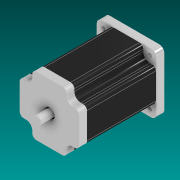
# Autodesk Inventor part: Nema 23 High toque
Saved by Autodesk Inventor 2020.3 (Build 243373000, 373)
## iProperties
Created: 2020-05-18
Part Number: Nema 23 High toque
Material: Aluminum 6061
Document SubType Name: Modeling
Designer: Svend
Density: 2.7 g/cm^3
Appearance: Aluminum - Polished
Author: Svend
Autodesk Inventor part; units mm, degrees
ref_plane "YZ Plane" through (0, 0, 0) normal (1, 0, 0) x (0, 1, 0)
ref_plane "XZ Plane" through (0, 0, 0) normal (0, 1, 0) x (-1, 0, 0)
ref_plane "XY Plane" through (0, 0, 0) normal (0, 0, 1) x (1, 0, 0)
sketch "Sketch1" plane through (0, 0, 0) normal (0, 0, 1) x (1, 0, 0)
  line L0 (24.95, 29.95) -> (-24.95, 29.95)
  line L1 (-29.95, 24.95) -> (-29.95, -24.95)
  line L2 (-24.95, -29.95) -> (24.95, -29.95)
  line L3 (29.95, -24.95) -> (29.95, 24.95)
  line L4 (29.95, 29.95) -> (-29.95, -29.95) construction
  line L5 (-29.95, 29.95) -> (29.95, -29.95) construction
  circle A0 centre (-23.57, 23.57) radius 2
  circle A1 centre (23.57, 23.57) radius 2
  circle A2 centre (23.57, -23.57) radius 2
  circle A3 centre (-23.57, -23.57) radius 2
  circle A4 centre (0, 0) radius 4.5
  arc A5 (-24.95, 29.95) -> (-29.95, 24.95) centre (-24.95, 24.95) ccw
  arc A6 (29.95, 24.95) -> (24.95, 29.95) centre (24.95, 24.95) ccw
  arc A7 (24.95, -29.95) -> (29.95, -24.95) centre (24.95, -24.95) ccw
  arc A8 (-29.95, -24.95) -> (-24.95, -29.95) centre (-24.95, -24.95) ccw
  dimension "d0" = 59.9
  dimension "d2" = 47.14
  dimension "d3" = 47.14
  dimension "d4" = 4
  dimension "d5" = 9
  dimension "d6" = 5
  dimension "d7" = 59.9
  dimension "d8" = 5
  dimension "d9" = 5
  constraints: 12 end point, 12 point on line, 9 centre point, 8 point on circle, 8 tangent, 4 equal radius, 2 horizontal alignment, 2 midpoint, 2 parallel, 1 coincident, 1 horizontal, 1 perpendicular
  measures "d0" distance of L5.end L4.end
  measures "d2" distance of A0.centre A1.centre
  measures "d3" distance of A2.centre A1.centre
  measures "d4" diameter of A0
  measures "d5" diameter of A4
  measures "d6" radius of A5
  measures "d7" distance between parallel lines of L2 L0
  measures "d8" radius of A6
  measures "d9" radius of A7
extrude "Extrusion1" add sketch "Sketch1" along normal blind 8
chamfer "Chamfer1" distance 0.5 angle 45 4 edges at (21.57, -23.57, 0) (-25.57, -23.57, 0) (21.57, 23.57, 0) (-25.57, 23.57, 0)
sketch "Sketch2" plane through (0, 0, 0) normal (0, 0, -1) x (-1, 0, 0)
  circle A0 centre (0, 0) radius 5 projected
  circle A1 centre (0, 0) radius 19
  circle A2 centre (0, 0) radius 4.5 projected
  dimension "d23" = 38
  constraints: 1 centre point, 1 coincident
  measures "d23" diameter of A1
extrude "Extrusion2" add sketch "Sketch2" along normal blind 2 contours A0 | A1
chamfer "Chamfer2" distance 0.5 angle 45 2 edges at (4.5, 0, -2) (19, 0, -2)
sketch "Sketch3" plane through (0, 0, 8) normal (0, 0, 1) x (1, 0, 0)
  arc A0 (24.95, -29.95) -> (29.95, -24.95) centre (24.95, -24.95) ccw projected
  line L0 (29.95, -24.95) -> (29.95, 24.95) projected
  arc A1 (29.95, 24.95) -> (24.95, 29.95) centre (24.95, 24.95) ccw projected
  line L1 (24.95, 29.95) -> (-24.95, 29.95) projected
  arc A2 (-24.95, 29.95) -> (-29.95, 24.95) centre (-24.95, 24.95) ccw projected
  line L2 (-29.95, 24.95) -> (-29.95, -24.95) projected
  arc A3 (-29.95, -24.95) -> (-24.95, -29.95) centre (-24.95, -24.95) ccw projected
  line L3 (-24.95, -29.95) -> (24.95, -29.95) projected
  circle A4 centre (0, 0) radius 4.5 projected
  circle A5 centre (-23.57, 23.57) radius 2 projected
  circle A6 centre (23.57, -23.57) radius 2 projected
  circle A7 centre (-23.57, -23.57) radius 2 projected
  circle A8 centre (23.57, 23.57) radius 2 projected
  circle A9 centre (-23.57, -23.57) radius 2 projected
  circle A10 centre (-23.57, -23.57) radius 6.38
  line L4 (-29.95, 24.95) -> (-29.95, -24.95) projected
  circle A11 centre (-23.57, 23.57) radius 2 projected
  circle A12 centre (-23.57, 23.57) radius 6.38
  line L5 (24.95, 29.95) -> (-24.95, 29.95) projected
  circle A13 centre (23.57, 23.57) radius 2 projected
  circle A14 centre (23.57, 23.57) radius 6.38
  circle A15 centre (23.57, -23.57) radius 6.38
  line L6 (-24.95, -29.95) -> (24.95, -29.95) projected
  line L7 (23.57, -17.19) -> (25.95, -17.19)
  line L8 (29.95, -24.95) -> (29.95, 24.95) projected
  line L9 (17.19, -23.57) -> (17.19, -25.95)
  line L10 (-17.19, -23.57) -> (-17.19, -25.95)
  line L11 (-23.57, -17.19) -> (-25.95, -17.19)
  line L12 (-23.57, 17.19) -> (-25.95, 17.19)
  line L13 (-17.19, 23.57) -> (-17.19, 25.95)
  line L14 (17.19, 23.57) -> (17.19, 25.95)
  line L15 (23.57, 17.19) -> (25.95, 17.19)
  line L16 (24.95, 29.95) -> (-24.95, 29.95) projected
  line L17 (29.95, -24.95) -> (29.95, 24.95) projected
  line L18 (-13.19, -29.95) -> (13.19, -29.95)
  line L19 (29.95, -13.19) -> (29.95, 13.19)
  line L20 (13.19, 29.95) -> (-13.19, 29.95)
  line L21 (-29.95, 13.19) -> (-29.95, -13.19)
  arc A16 (-29.95, -13.19) -> (-25.95, -17.19) centre (-25.95, -13.19) ccw
  arc A17 (-25.95, 17.19) -> (-29.95, 13.19) centre (-25.95, 13.19) ccw
  arc A18 (-13.19, 29.95) -> (-17.19, 25.95) centre (-13.19, 25.95) ccw
  arc A19 (17.19, 25.95) -> (13.19, 29.95) centre (13.19, 25.95) ccw
  arc A20 (29.95, 13.19) -> (25.95, 17.19) centre (25.95, 13.19) ccw
  arc A21 (25.95, -17.19) -> (29.95, -13.19) centre (25.95, -13.19) ccw
  arc A22 (13.19, -29.95) -> (17.19, -25.95) centre (13.19, -25.95) ccw
  arc A23 (-17.19, -25.95) -> (-13.19, -29.95) centre (-13.19, -25.95) ccw
  point P0 (29.95, -17.19)
  point P1 (17.19, -29.95)
  point P2 (-17.19, -29.95)
  point P3 (-29.95, -17.19)
  point P4 (-29.95, 17.19)
  point P5 (-17.19, 29.95)
  point P6 (17.19, 29.95)
  point P7 (29.95, 17.19)
  point P8 (29.95, 13.19)
  dimension "d29" = 4
  dimension "d30" = 4
  constraints: 28 tangent, 24 end point, 24 point on circle, 24 point on line, 12 centre point, 7 parallel, 6 equal radius, 6 perpendicular, 4 coincident, 3 collinear, 2 horizontal, 1 vertical
  measures "d29" radius of A16
  measures "d30" radius of A23
extrude "Extrusion3" add sketch "Sketch3" along normal blind 70 contours L3 A23 L10 A10 L11 A16 L2 A17 L12 A12 L13 A18 L1 A19 L14 A14 L15 A20 L0 A21 L7 A15 L9 A22
sketch "Sketch5" plane through (0, 0, 78) normal (0, 0, 1) x (1, 0, 0)
  arc A0 (17.19, 23.57) -> (23.57, 17.19) centre (23.57, 23.57) ccw projected
  line L0 (17.19, 23.57) -> (17.19, 25.95) projected
  arc A1 (17.19, 25.95) -> (13.19, 29.95) centre (13.19, 25.95) ccw projected
  line L1 (13.19, 29.95) -> (-13.19, 29.95) projected
  arc A2 (-13.19, 29.95) -> (-17.19, 25.95) centre (-13.19, 25.95) ccw projected
  line L2 (-17.19, 25.95) -> (-17.19, 23.57) projected
  arc A3 (-23.57, 17.19) -> (-17.19, 23.57) centre (-23.57, 23.57) ccw projected
  line L3 (-23.57, 17.19) -> (-25.95, 17.19) projected
  arc A4 (-25.95, 17.19) -> (-29.95, 13.19) centre (-25.95, 13.19) ccw projected
  line L4 (-29.95, 13.19) -> (-29.95, -13.19) projected
  arc A5 (-29.95, -13.19) -> (-25.95, -17.19) centre (-25.95, -13.19) ccw projected
  line L5 (-25.95, -17.19) -> (-23.57, -17.19) projected
  arc A6 (-17.19, -23.57) -> (-23.57, -17.19) centre (-23.57, -23.57) ccw projected
  line L6 (-17.19, -23.57) -> (-17.19, -25.95) projected
  arc A7 (-17.19, -25.95) -> (-13.19, -29.95) centre (-13.19, -25.95) ccw projected
  line L7 (-13.19, -29.95) -> (13.19, -29.95) projected
  arc A8 (13.19, -29.95) -> (17.19, -25.95) centre (13.19, -25.95) ccw projected
  line L8 (17.19, -25.95) -> (17.19, -23.57) projected
  arc A9 (23.57, -17.19) -> (17.19, -23.57) centre (23.57, -23.57) ccw projected
  line L9 (23.57, -17.19) -> (25.95, -17.19) projected
  arc A10 (25.95, -17.19) -> (29.95, -13.19) centre (25.95, -13.19) ccw projected
  line L10 (29.95, -13.19) -> (29.95, 13.19) projected
  arc A11 (29.95, 13.19) -> (25.95, 17.19) centre (25.95, 13.19) ccw projected
  line L11 (25.95, 17.19) -> (23.57, 17.19) projected
  circle A12 centre (0, 0) radius 4.5 projected
  line L12 (-23.57, -17) -> (-25.95, -17)
  arc A13 (-29.76, -13.19) -> (-25.95, -17) centre (-25.95, -13.19) ccw
  line L13 (-29.76, -13.19) -> (-29.76, 13.19)
  arc A14 (-25.95, 17) -> (-29.76, 13.19) centre (-25.95, 13.19) ccw
  line L14 (-25.95, 17) -> (-23.57, 17)
  arc A15 (-23.57, 17) -> (-17, 23.57) centre (-23.57, 23.57) ccw
  line L15 (-17, 23.57) -> (-17, 25.95)
  arc A16 (-13.19, 29.76) -> (-17, 25.95) centre (-13.19, 25.95) ccw
  line L16 (-13.19, 29.76) -> (13.19, 29.76)
  arc A17 (17, 25.95) -> (13.19, 29.76) centre (13.19, 25.95) ccw
  line L17 (17, 25.95) -> (17, 23.57)
  arc A18 (17, 23.57) -> (23.57, 17) centre (23.57, 23.57) ccw
  line L18 (23.57, 17) -> (25.95, 17)
  arc A19 (29.76, 13.19) -> (25.95, 17) centre (25.95, 13.19) ccw
  line L19 (29.76, 13.19) -> (29.76, -13.19)
  arc A20 (25.95, -17) -> (29.76, -13.19) centre (25.95, -13.19) ccw
  line L20 (25.95, -17) -> (23.57, -17)
  arc A21 (23.57, -17) -> (17, -23.57) centre (23.57, -23.57) ccw
  line L21 (17, -23.57) -> (17, -25.95)
  arc A22 (13.19, -29.76) -> (17, -25.95) centre (13.19, -25.95) ccw
  line L22 (13.19, -29.76) -> (-13.19, -29.76)
  arc A23 (-17, -25.95) -> (-13.19, -29.76) centre (-13.19, -25.95) ccw
  line L23 (-17, -25.95) -> (-17, -23.57)
  arc A24 (-17, -23.57) -> (-23.57, -17) centre (-23.57, -23.57) ccw
  dimension "d38" = 0.19
  constraints: 24 end point, 24 point on circle, 12 centre point, 23 other
  measures "d38" distance between parallel lines of L5 L12
extrude "Extrusion6" cut sketch "Sketch5" against normal up to surface (70 mm away) contours A0 L11 A11 L10 A10 L9 A9 L8 A8 L7 A7 L6 A6 L5 A5 L4 A4 L3 A3 L2 A2 L1 A1 L0
sketch "Sketch6" plane through (0, 0, 78) normal (0, 0, 1) x (1, 0, 0)
  line L0 (25.95, 17) -> (23.57, 17) projected
  arc A0 (17, 23.57) -> (23.57, 17) centre (23.57, 23.57) ccw projected
  line L1 (17, 23.57) -> (17, 25.95) projected
  arc A1 (17, 25.95) -> (13.19, 29.76) centre (13.19, 25.95) ccw projected
  line L2 (13.19, 29.76) -> (-13.19, 29.76) projected
  arc A2 (-13.19, 29.76) -> (-17, 25.95) centre (-13.19, 25.95) ccw projected
  line L3 (-17, 25.95) -> (-17, 23.57) projected
  arc A3 (-23.57, 17) -> (-17, 23.57) centre (-23.57, 23.57) ccw projected
  line L4 (-23.57, 17) -> (-25.95, 17) projected
  arc A4 (-25.95, 17) -> (-29.76, 13.19) centre (-25.95, 13.19) ccw projected
  line L5 (-29.76, 13.19) -> (-29.76, -13.19) projected
  arc A5 (-29.76, -13.19) -> (-25.95, -17) centre (-25.95, -13.19) ccw projected
  line L6 (-25.95, -17) -> (-23.57, -17) projected
  arc A6 (-17, -23.57) -> (-23.57, -17) centre (-23.57, -23.57) ccw projected
  line L7 (-17, -23.57) -> (-17, -25.95) projected
  arc A7 (-17, -25.95) -> (-13.19, -29.76) centre (-13.19, -25.95) ccw projected
  line L8 (-13.19, -29.76) -> (13.19, -29.76) projected
  arc A8 (13.19, -29.76) -> (17, -25.95) centre (13.19, -25.95) ccw projected
  line L9 (17, -25.95) -> (17, -23.57) projected
  arc A9 (23.57, -17) -> (17, -23.57) centre (23.57, -23.57) ccw projected
  line L10 (23.57, -17) -> (25.95, -17) projected
  arc A10 (25.95, -17) -> (29.76, -13.19) centre (25.95, -13.19) ccw projected
  line L11 (29.76, -13.19) -> (29.76, 13.19) projected
  arc A11 (29.76, 13.19) -> (25.95, 17) centre (25.95, 13.19) ccw projected
  circle A12 centre (0, 0) radius 4.5 projected
  arc A13 (-29.902, -13.19) -> (-25.95, -17.142) centre (-25.95, -13.19) ccw
  line L12 (-29.902, -13.19) -> (-29.902, 13.19)
  arc A14 (-25.95, 17.142) -> (-29.902, 13.19) centre (-25.95, 13.19) ccw
  line L13 (-25.95, 17.142) -> (-23.57, 17.142)
  arc A15 (-23.57, 17.142) -> (-17.142, 23.57) centre (-23.57, 23.57) ccw
  line L14 (-17.142, 23.57) -> (-17.142, 25.95)
  arc A16 (-13.19, 29.902) -> (-17.142, 25.95) centre (-13.19, 25.95) ccw
  line L15 (-13.19, 29.902) -> (13.19, 29.902)
  arc A17 (17.142, 25.95) -> (13.19, 29.902) centre (13.19, 25.95) ccw
  line L16 (17.142, 25.95) -> (17.142, 23.57)
  arc A18 (17.142, 23.57) -> (23.57, 17.142) centre (23.57, 23.57) ccw
  line L17 (23.57, 17.142) -> (25.95, 17.142)
  arc A19 (29.902, 13.19) -> (25.95, 17.142) centre (25.95, 13.19) ccw
  line L18 (29.902, 13.19) -> (29.902, -13.19)
  arc A20 (25.95, -17.142) -> (29.902, -13.19) centre (25.95, -13.19) ccw
  line L19 (25.95, -17.142) -> (23.57, -17.142)
  arc A21 (23.57, -17.142) -> (17.142, -23.57) centre (23.57, -23.57) ccw
  line L20 (17.142, -23.57) -> (17.142, -25.95)
  arc A22 (13.19, -29.902) -> (17.142, -25.95) centre (13.19, -25.95) ccw
  line L21 (13.19, -29.902) -> (-13.19, -29.902)
  arc A23 (-17.142, -25.95) -> (-13.19, -29.902) centre (-13.19, -25.95) ccw
  line L22 (-17.142, -25.95) -> (-17.142, -23.57)
  arc A24 (-17.142, -23.57) -> (-23.57, -17.142) centre (-23.57, -23.57) ccw
  line L23 (-23.57, -17.142) -> (-25.95, -17.142)
  dimension "d41" = 0.142
  constraints: 24 end point, 24 point on circle, 12 centre point, 23 other
  measures "d41" radial gap between concentric circles of A5 A13
extrude "Extrusion7" add sketch "Sketch6" along normal blind 8 contours A11 L11 A10 L10 A9 L9 A8 L8 A7 L7 A6 L6 A5 L5 A4 L4 A3 L3 A2 L2 A1 L1 A0 L0 | L12 A14 L13 A15 L14 A16 L15 A17 L16 A18 L17 A19 L18 A20 L19 A21 L20 A22 L21 A23 L22 A24 L23 A13
sketch "Sketch7" plane through (0, 0, 86) normal (0, 0, 1) x (1, 0, 0)
  circle A0 centre (0, 0) radius 4.5 projected
  circle A1 centre (0, 0) radius 4
  dimension "d55" = 8
  constraints: 1 centre point, 1 coincident
  measures "d55" diameter of A1
extrude "Extrusion8" add sketch "Sketch7" along normal blind 13 and the other way blind 95 contours A1
sketch "Sketch8" plane through (0, 0, -2) normal (0, 0, -1) x (-1, 0, 0)
  circle A0 centre (0, 0) radius 4.5 projected
  circle A1 centre (0, 0) radius 5 projected
extrude "Extrusion9" cut sketch "Sketch8" against normal blind 10
sketch "Sketch9" plane through (0, 0, 86) normal (0, 0, 1) x (1, 0, 0)
  circle A0 centre (0, 0) radius 4.5 projected
  circle A1 centre (0, 0) radius 5 projected
extrude "Extrusion10" cut sketch "Sketch9" against normal blind 10
chamfer "Chamfer3" distance 0.5 angle 45 4 edges at (-5, 0, 86) (5, 0, -2) (-4, 0, -9) (-4, 0, 99)
equation "\"d3\" = d2"
equation "\"d7\" = d0"
body "Solid1"
